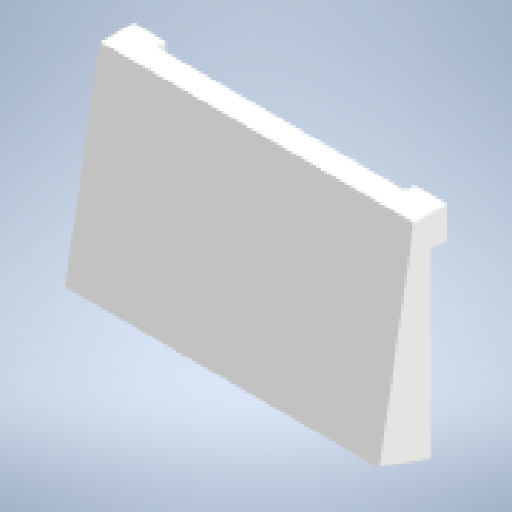
# Autodesk Inventor part: Display Case
Saved by Autodesk Inventor 2024 (Build 280153000, 153)
## iProperties
Created: 2024-10-16
Part Number: Display Case
Material: ABS Plastic
Document SubType Name: Modeling
Designer: Ishaan
Density: 1.06 g/cm^3
Appearance: Smooth - White
Author: Ishaan
Autodesk Inventor part; units mm, degrees
ref_plane "YZ Plane" through (0, 0, 0) normal (1, 0, 0) x (0, 1, 0)
ref_plane "XZ Plane" through (0, 0, 0) normal (0, 1, 0) x (-1, 0, 0)
sketch "Sketch1" plane through (0, 0, 0) normal (0, 0, 1) x (1, 0, 0)
  line L0 (-75, -10) -> (-95, -10)
  line L1 (-95, -10) -> (-95, 10)
  line L2 (-95, 10) -> (-75, 10)
  line L3 (-75, 10) -> (-75, -10)
  line L4 (-75, -10) -> (-95, 10) construction
  line L5 (-95, -10) -> (-75, 10) construction
  line L6 (95, -10) -> (75, -10)
  line L7 (75, -10) -> (75, 10)
  line L8 (75, 10) -> (95, 10)
  line L9 (95, 10) -> (95, -10)
  line L10 (95, -10) -> (75, 10) construction
  line L11 (75, -10) -> (95, 10) construction
  line L12 (-85, 0) -> (85, 0) construction
  point P0 (0, 0)
  point P1 (0, 0)
  dimension "d0" = 20
  dimension "d1" = 20
  dimension "d2" = 20
  dimension "d3" = 20
  dimension "d4" = 170
  constraints: 26 end point, 5 midpoint, 4 parallel, 3 horizontal, 2 perpendicular, 1 coincident
  measures "d0" distance of L1.end L2.end
  measures "d1" distance of L0.end L1.end
  measures "d2" distance of L7.end L8.end
  measures "d3" distance of L6.end L7.end
  measures "d4" distance of L12.start L12.end
extrude "Extrusion1" add sketch "Sketch1" along normal blind 5
sketch "Sketch2" plane through (0, 0, 5) normal (0, 0, 1) x (1, 0, 0)
  line L0 (-75, 10) -> (-95, 10) projected
  line L1 (-95, 10) -> (-95, -10) projected
  line L2 (-95, -10) -> (-75, -10) projected
  line L3 (-75, -10) -> (-75, 10) projected
  line L4 (95, 10) -> (75, 10) projected
  line L5 (75, 10) -> (75, -10) projected
  line L6 (75, -10) -> (95, -10) projected
  line L7 (95, -10) -> (95, 10) projected
  line L8 (-95, 10) -> (95, 10)
  line L9 (95, 10) -> (95, -10)
  line L10 (95, -10) -> (-95, -10)
  line L11 (-95, -10) -> (-95, 10)
  point P0 (0, 0)
  constraints: 8 end point, 2 parallel, 1 horizontal, 1 perpendicular
extrude "Extrusion2" add sketch "Sketch2" along normal blind 5
ref_plane "Work Plane1" through (75, 5.75, 0) normal (0, 1, 0) x (1, 0, 0)
sketch "Sketch4" plane through (95, -10, 0) normal (1, 0, 0) x (0, 0, -1)
  line L0 (0, 0) -> (0, 20) projected
  line L1 (0, 20) -> (-10, 20) projected
  line L2 (-10, 0) -> (-10, 20) projected
  line L3 (0, 0) -> (-10, 0) projected
  line L4 (-10, 20) -> (-20, 20)
  line L5 (-20, 20) -> (-40.8378, -98.1769)
  line L6 (-40.8378, -98.1769) -> (-10, -109.401)
  line L7 (0, 0) -> (0, 20) projected
  line L8 (-10, -109.401) -> (-10, 0)
  line L9 (-10, 0) -> (-10, 20) projected
  point P0 (0, 10)
  dimension "d14" = 100
  dimension "d15" = 100
  dimension "d16" = 120
  dimension "d17" = 20
  constraints: 8 end point, 1 collinear, 1 horizontal
  measures "d14" angle of L4 L5
  measures "d15" angle of L6 L5
  measures "d16" distance of L4.end L5.end
  measures "d17" distance from line of L0 L4.end
extrude "Extrusion4" add sketch "Sketch4" against normal up to surface (190 mm away) contours L8 L6 L5 L4 L2
fillet "Fillet1" radius 2 2 edges at (-75, 0, 5) (75, 0, 5)
fillet "Fillet2" radius 1 9 edges at (-75, 10, 1.5) (75, 10, 1.5) (-75, -10, 1.5) (75, -10, 1.5) (95, -10, 5) (95, 10, 10) (-95, 10, 10) (-95, -10, 5) (95, -113.7889, 25.4189)
equation "\"d15\" = d14"
body "Solid1"
